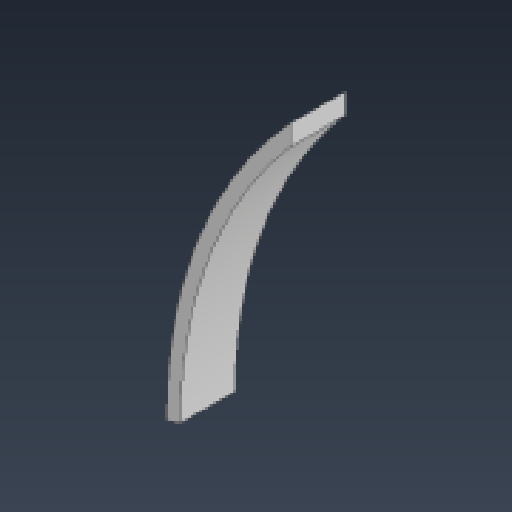
# Autodesk Inventor part: направление
Saved by Autodesk Inventor 2025 (Build 290162000, 162)
## iProperties
Created: 2025-11-04
Part Number: направление
Material: Типовые
Document SubType Name: Modeling
Designer: GameHD
Density: 1 g/cm^3
Appearance: По умолчанию
Author: GameHD
Autodesk Inventor part; units mm, degrees
ref_plane "YZ Plane" through (0, 0, 0) normal (1, 0, 0) x (0, 1, 0)
ref_plane "XZ Plane" through (0, 0, 0) normal (0, 1, 0) x (-1, 0, 0)
ref_plane "XY Plane" through (0, 0, 0) normal (0, 0, 1) x (1, 0, 0)
sketch "Эскиз1" plane through (0, 0, 0) normal (0, 0, 1) x (1, 0, 0)
  circle A0 centre (0, 0) radius 166
  circle A1 centre (0, 0) radius 170.5
  line L0 (-126, 0) -> (-124.8304, 116.1363)
  line L1 (-131.4755, 117.5684) -> (-196.563, 74.7059)
  line L2 (-166, 0) -> (-154.6003, 3.748)
  line L3 (-166, 0) -> (-154, 0) construction
  line L4 (-166, 0) -> (-170.4936, -1.4774)
  point P0 (-170.5, 0)
  point P1 (-124.8988, 109.3449)
  point P2 (-123, 114.4334)
  dimension "d0" = 332
  dimension "d1" = 341
  dimension "d2" = 40
  dimension "d5" = 12
  dimension "d6" = 18.2
  constraints: 10 end point, 3 point on circle, 2 coincident, 1 centre point, 1 collinear, 1 equal length, 1 horizontal, 1 tangent, 3 other
  measures "d1" diameter of A1
  measures "d2" distance of L2.start L0.start
  measures "d5" distance of L2.start L2.end
  measures "d6" angle of L3 L2
extrude "Выдавливание1" add sketch "Эскиз1" along normal blind 20 contours L4 A1 L0 A0 picked at (-167.2026, 23.0577)
